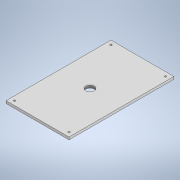
# Autodesk Inventor part: top
Saved by Autodesk Inventor 2020 (Build 240168000, 168)
## iProperties
Created: 2019-11-30
Part Number: top
Material: Générique
Document SubType Name: Modeling
Designer: bapti
Density: 1 g/cm^3
Appearance: Par défaut
Author: bapti
Autodesk Inventor part; units mm, degrees
ref_plane "YZ Plane" through (0, 0, 0) normal (1, 0, 0) x (0, 1, 0)
ref_plane "XZ Plane" through (0, 0, 0) normal (0, 1, 0) x (-1, 0, 0)
ref_plane "XY Plane" through (0, 0, 0) normal (0, 0, 1) x (1, 0, 0)
sketch "Esquisse1" plane through (0, 0, 0) normal (0, 1, 0) x (-1, 0, 0)
  line L0 (0, 0) -> (150, 0)
  line L1 (150, 0) -> (150, -250)
  line L2 (150, -250) -> (0, -250)
  line L3 (0, -250) -> (0, 0)
  line L4 (0, 0) -> (150, -250) construction
  line L5 (0, -250) -> (150, 0) construction
  circle A0 centre (75, -125) radius 10
  circle A1 centre (140, -10) radius 2.1
  line L6 (140, -10) -> (150, -10) construction
  line L7 (140, -10) -> (140, 0) construction
  line L8 (0, -125) -> (150, -125) construction
  line L9 (75, 0) -> (75, -250) construction
  circle A2 centre (10, -10) radius 2.1
  circle A3 centre (140, -240) radius 2.1
  circle A4 centre (10, -240) radius 2.1
  dimension "d0" = 150
  dimension "d1" = 250
  dimension "d2" = 20
  dimension "d5" = 4.2
  dimension "d7" = 10
  constraints: 20 end point, 5 centre point, 5 midpoint, 4 perpendicular, 3 symmetric about line, 2 parallel, 2 point on line, 1 horizontal, 3 other
  measures "d0" distance of L1.end L2.end
  measures "d1" distance of L2.end L0.start
  measures "d2" diameter of A0
  measures "d5" diameter of A1
  measures "d7" distance of L6.start L6.end
extrude "Extrusion1" add sketch "Esquisse1" along normal blind 6
